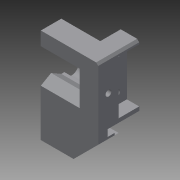
# Autodesk Inventor part: switchlock1l
Saved by Autodesk Inventor 2015 (Build 190159000, 159)
## iProperties
Created: 2020-08-08
Part Number: switchlock1l
Material: 일반
Document SubType Name: Modeling
Designer: penta
Density: 1 g/cm^3
Appearance: 기본값
Author: penta
Autodesk Inventor part; units mm, degrees
ref_plane "YZ Plane" through (0, 0, 0) normal (1, 0, 0) x (0, 1, 0)
ref_plane "XZ Plane" through (0, 0, 0) normal (0, 1, 0) x (-1, 0, 0)
ref_plane "XY Plane" through (0, 0, 0) normal (0, 0, 1) x (1, 0, 0)
sketch "스케치3" plane through (0, 0, 0) normal (0, 1, 0) x (-1, 0, 0)
  line L0 (0, 0) -> (9, 0)
  line L1 (9, 0) -> (9, -30)
  line L2 (9, -30) -> (0, -30)
  line L3 (0, -30) -> (0, 0)
  dimension "d26" = 9
  dimension "d27" = 30
  constraints: 8 end point, 2 parallel, 1 horizontal, 1 perpendicular
  measures "d26" distance of L1.end L2.end
  measures "d27" distance of L0.end L1.end
extrude "돌출3" add sketch "스케치3" along normal blind 10
sketch "스케치4" plane through (0, 10, 0) normal (0, 1, 0) x (1, 0, 0)
  line L0 (0, 0) -> (0, 30) projected
  line L1 (0, 2) -> (-6, 2)
  line L2 (-6, 2) -> (-6, 28)
  line L3 (-6, 28) -> (0, 28)
  line L4 (0, 28) -> (0, 2)
  line L5 (0, 0) -> (-9, 0)
  line L6 (-9, 0) -> (-9, 30)
  line L7 (-9, 30) -> (0, 30)
  line L8 (0, 30) -> (0, 0)
  dimension "d30" = 6
  dimension "d31" = 26
  constraints: 16 end point, 4 parallel, 2 horizontal, 2 perpendicular, 1 point on line
  measures "d30" distance of L2.end L3.end
  measures "d31" distance of L1.end L2.end
extrude "돌출4" add sketch "스케치4" along normal blind 10 contours L5 L6 L7 L0 L3 L2 L1
hole "구멍3" at (-9, 15, -7) direction (1, 0, 0) diameter 3.25 end through all
hole "구멍6" at (0, 5, -15) direction (-1, 0, 0) diameter 2.85 end through all
sketch "스케치7" plane through (-9, 0, -30) normal (-1, 0, 0) x (0, 0, 1)
  line L0 (0, 0) -> (6.8868, 0)
  line L1 (30, 0) -> (30, 10)
  line L2 (30, 10) -> (23.1132, 10)
  line L3 (0, 10) -> (0, 0)
  line L4 (0, 5) -> (30, 5)
  line L5 (28, 10) -> (2, 10) projected
  line L6 (6.8868, 10) -> (9.7735, 5)
  line L7 (9.7735, 5) -> (6.8868, 0)
  line L8 (6.8868, 0) -> (1.1132, 0)
  line L9 (1.1132, 10) -> (6.8868, 10)
  line L10 (28.8868, 0) -> (23.1132, 0)
  line L11 (23.1132, 0) -> (20.2265, 5)
  line L12 (20.2265, 5) -> (23.1132, 10)
  line L13 (23.1132, 10) -> (28.8868, 10)
  line L14 (6.8868, 0) -> (23.1132, 0)
  line L15 (6.8868, 10) -> (0, 10)
  line L16 (23.1132, 10) -> (6.8868, 10)
  line L17 (23.1132, 0) -> (30, 0)
  point P0 (4, 5)
  point P1 (26, 5)
  point P2 (4, 5)
  point P3 (4, 10)
  point P4 (26, 5)
  point P5 (26, 10)
  constraints: 34 end point, 10 parallel, 4 midpoint, 4 point on line, 3 horizontal, 3 perpendicular, 2 coincident, 16 other
extrude "돌출7" add sketch "스케치7" along normal blind 19 contours L3 L4 L7 L0 | L3 L15 L9 L5 L6 L4 | L11 L4 L1 L17 L10 | L12 L2 L1 L4
thicken "두껍게 하기1" operation add thickness 0.1 both sides no extend neighbours yes toward (0, 0, -1) faces at (-2, 13.3333, -28) (-4, 13.3333, -2)
thicken "두껍게 하기2" operation add thickness 0.2 both sides no extend neighbours yes toward (0, -0.5, 0.8660254) faces at (-15.3333, 8.3333, -7.849) (-15.3333, 3.3333, -8.8113) (-15.3333, 6.6667, -21.1887) (-15.3333, 1.6667, -22.151)
hole "구멍8" at (-9, 15, -23) direction (1, 0, 0) diameter 3.25 end through all
sketch "스케치15" plane through (0, 0, 0) normal (1, 0, 0) x (0, 0, -1)
  line L0 (23.3442, 0) -> (30, 0)
  line L1 (30, 0) -> (30, 20)
  line L2 (30, 20) -> (23.3442, 20)
  line L3 (23.3442, 20) -> (23.3442, 0)
  constraints: 8 end point, 2 parallel, 1 horizontal, 1 perpendicular
extrude "돌출12" add sketch "스케치15" against normal up to surface (19 mm away) from surface at -9
hole "구멍9" at (-28, 15, -23) direction (1, 0, 0) diameter 7 depth 19
sketch "스케치16" plane through (0, 0, 0) normal (1, 0, 0) x (0, 0, -1)
  line L0 (30, 0) -> (33.3, 0)
  line L1 (33.3, 5) -> (30, 5)
  line L2 (30, 5) -> (30, 0)
  line L3 (33.3, 0) -> (36.3, 0)
  line L4 (36.3, 8) -> (33.3, 8)
  line L5 (33.3, 8) -> (33.3, 5)
  line L6 (46.3, 0) -> (36.3, 0)
  line L7 (46.3, 20) -> (46.3, 0)
  line L8 (44.3, 20) -> (44.3, 8)
  line L9 (44.3, 8) -> (36.3, 8)
  line L10 (44.3, 20) -> (46.3, 20)
  point P0 (0, 0)
  dimension "d161" = 3.3
  dimension "d162" = 5
  dimension "d163" = 3
  dimension "d164" = 8
  constraints: 22 end point, 3 horizontal, 3 parallel, 1 perpendicular, 1 vertical
  measures "d161" distance of L1.end L1.start
  measures "d162" distance of L1.start L0.end
  measures "d163" distance of L4.end L4.start
  measures "d164" distance of L3.end L4.start
extrude "돌출13" add sketch "스케치16" against normal up to surface (28 mm away)
hole "구멍10" at (-16, 14, -23.3442) direction (0, 0, -1) diameter 2.85 end up to face face through (-18.6667, 13.3333, -46.3) facing (0, 0, -1) counterbore diameter 7 counterbore depth 4
thicken "두껍게 하기3" operation add thickness 0.4 both sides no extend neighbours yes toward (0, -1, 0) faces at (-18.6667, 5, -32.2)
chamfer "모따기1" distance 1 angle 45 1 edges at (0, 10, 0)
chamfer "모따기4" distance 12 angle 45 1 edges at (0, 10, -46.3)
